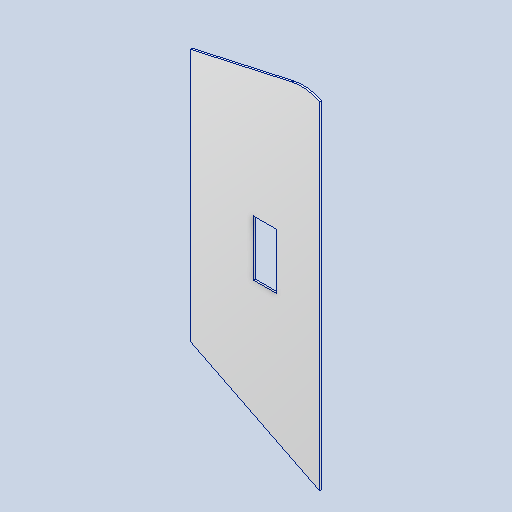
# Autodesk Inventor part: pokrywa lewa
Saved by Autodesk Inventor 2023 (Build 270158000, 158)
## iProperties
Created: 2022-10-11
Part Number: pokrywa lewa
Material: Aluminum 6061
Document SubType Name: Modeling
Designer: komputer
Density: 2.7 g/cm^3
Appearance: Aluminum - Flat
Author: komputer
Autodesk Inventor part; units mm, degrees
ref_plane "YZ Plane" through (0, 0, 0) normal (1, 0, 0) x (0, 1, 0)
ref_plane "XZ Plane" through (0, 0, 0) normal (0, 1, 0) x (-1, 0, 0)
ref_plane "XY Plane" through (0, 0, 0) normal (0, 0, 1) x (1, 0, 0)
sketch "Sketch1" plane through (0, 0, 0) normal (0, 0, 1) x (1, 0, 0)
  line L0 (7.5, 3.8038) -> (3.6225, 3.8038) projected
  arc A0 (1.9153, 4.762) -> (3.6225, 3.8038) centre (3.6225, 5.8038) ccw projected
  line L1 (1.9153, 4.762) -> (-2.2072, 11.517) projected
  arc A1 (-2.5, 12.5588) -> (-2.2072, 11.517) centre (-0.5, 12.5588) ccw projected
  line L2 (-2.5, 12.5588) -> (-2.5, 21.8038) projected
  arc A2 (-0.5, 23.8038) -> (-2.5, 21.8038) centre (-0.5, 21.8038) ccw projected
  line L3 (-0.5, 23.8038) -> (7.5, 23.8038) projected
  line L4 (7.5, 23.8038) -> (7.5, 3.8038) projected
  spline S0 degree 3 poles (-6.0485, -11.2843) (-6.0213, -11.0209) (-5.9428, -10.7653) (-5.6929, -10.2997) (-5.524, -10.094) (-5.1467, -9.7842) (-4.9505, -9.6718) (-4.5292, -9.5173) (-4.3073, -9.4763) (-4.0832, -9.4731) knots 0 0 0 0 0.079442 0.079442 0.158531 0.158531 0.225919 0.225919 0.293184 0.293184 0.293184 0.293184 projected
  line L5 (-6.0485, -11.2843) -> (-6.563, -16.2598) projected
  line L6 (-6.563, -16.2598) -> (-6.8849, -19.6266) projected
  arc A3 (-6.8849, -19.6266) -> (-5.7884, -21.6058) centre (-4.894, -19.817) ccw projected
  line L7 (17.5, -33.2499) -> (-5.7884, -21.6058) projected
  line L8 (17.5, 31.9794) -> (17.5, -33.2499) projected
  arc A4 (4.376, 33.2499) -> (17.5, 31.9794) centre (12.5, 48.7499) ccw projected
  arc A5 (-1.8324, 56.2463) -> (4.376, 33.2499) centre (12.5, 47.7794) ccw projected
  line L9 (-1.8324, 56.2463) -> (-17.5, 52.7794) projected
  line L10 (-17.5, 52.7794) -> (-17.5, 3.0185) projected
  ellipse E0 centre (-15.5, 3.0185) end of major axis (-15.5, 1.0011) minor radius 2 (-17.5, 3.0185) -> (-15.6888, 1.0101) ccw projected
  line L11 (-15.6888, 1.0101) -> (-3.1949, -0.1848) projected
  line L12 (-3.1949, -0.1848) -> (-4.0832, -9.4731) projected
  circle A6 centre (-12, 26.728) radius 1.25 projected
  circle A7 centre (5.3255, 26.728) radius 1.25 projected
  line L13 (-14, 9.2999) -> (-10, 9.2999) projected
  line L14 (-14, 15.6999) -> (-14, 9.2999) projected
  line L15 (-10, 15.6999) -> (-14, 15.6999) projected
  line L16 (-10, 9.2999) -> (-10, 15.6999) projected
  line L17 (13.7851, 6.0601) -> (9.7851, 6.0601) projected
  line L18 (13.7851, -0.3399) -> (13.7851, 6.0601) projected
  line L19 (9.7851, -0.3399) -> (13.7851, -0.3399) projected
  line L20 (9.7851, 6.0601) -> (9.7851, -0.3399) projected
  circle A8 centre (7.1425, -8.6154) radius 1.25 projected
  line L21 (17.5, -33.2499) -> (-17.5, -15.7501) projected
  line L22 (-17.5, -15.7501) -> (-17.5, -17.9862) projected
  line L23 (-17.5, -17.9862) -> (17.5, -35.486) projected
  line L24 (17.5, -35.486) -> (17.5, -33.2499) projected
  line L25 (-1.4649, 56.8397) -> (-18, 53.1809) projected
  line L26 (-18, 53.1809) -> (-18, -17.9862) projected
  line L27 (-18, -17.9862) -> (-17.5, -17.9862) projected
  line L28 (-17.5, -17.9862) -> (-17.5, 52.7794) projected
  line L29 (-17.5, 52.7794) -> (-1.8324, 56.2463) projected
  arc A9 (-1.4649, 56.8397) -> (-1.8324, 56.2463) centre (12.5, 47.7794) ccw projected
  line L30 (19.5, -37.0206) -> (19.5, 31.9794) projected
  line L31 (19.5, 31.9794) -> (17.5, 31.9794) projected
  line L32 (17.5, -37.0206) -> (17.5, 31.9794) projected
  line L33 (19.5, -37.0206) -> (17.5, -37.0206) projected
  circle A10 centre (12.5, 47.7794) radius 15.02 projected
  line L34 (-1.4649, 56.8397) -> (-11.9805, 54.5129)
  line L35 (-11.9805, 54.5129) -> (26.5324, 63.5095)
  line L36 (17.5, 31.9794) -> (17.5, 20.7849)
  line L37 (17.5, 20.7849) -> (17.5, 78.444)
  circle A11 centre (12.5, 47.7794) radius 12.1257
  line L38 (-17.5, -15.7501) -> (-17.5, 52.7794)
  line L39 (-1.8324, 56.2463) -> (11.2654, 59.1445)
  line L40 (11.2654, 59.1445) -> (26.5324, 62.5227)
  circle A12 centre (12.5, 47.7794) radius 11.3634
  line L41 (5.8925, 7.1892) -> (-0.5, 7.1892)
  line L42 (-0.5, 7.1892) -> (-0.5, 22.231)
  line L43 (-0.5, 22.231) -> (5.8925, 22.231)
  line L44 (5.8925, 22.231) -> (5.8925, 7.1892)
  point P0 (0, 0)
  point P1 (17.5, 57.9837)
  point P2 (10.0449, 58.8745)
  constraints: 22 end point, 4 point on line, 2 centre point, 2 coincident, 2 parallel, 2 tangent, 1 collinear, 1 horizontal, 1 perpendicular, 1 other
extrude "Extrusion1" add sketch "Sketch1" along normal blind 0.5 contours L0 A0 L1 L41 L44 L43 L42 A1 L2 A2 L3 L4 | L5 L6 A3 L21 L28 E0 L11 L12 S0 | S0 L12 L11 E0 L10 L9 A5 A4 L8 L7 A3 L6 L5 | L39 A10 L37 A4 A5 | L39 A11 L37 A10 | L39 A12 L37 A11 | A12 L37 | L14 L15 L16 L13 | L18 L19 L20 L17 picked at (9.8401, 51.5561)
sketch "Sketch2" plane through (0, 0, 0.5) normal (0, 0, 1) x (1, 0, 0)
  line L0 (17.5, -33.2499) -> (17.5, 57.9837) projected
  arc A0 (17.5, 57.9837) -> (10.0449, 58.8745) centre (12.5, 47.7794) ccw projected
  line L1 (10.0449, 58.8745) -> (-17.5, 52.7794) projected
  line L2 (-17.5, 52.7794) -> (-17.5, -15.7501) projected
  line L3 (-17.5, -15.7501) -> (17.5, -33.2499) projected
  circle A1 centre (-12, 26.728) radius 1.25 projected
  circle A2 centre (5.3255, 26.728) radius 1.25 projected
  circle A3 centre (7.1425, -8.6154) radius 1.25 projected
  line L4 (-0.5, 7.1892) -> (-0.5, 22.231) projected
  line L5 (-0.5, 22.231) -> (5.8925, 22.231) projected
  line L6 (5.8925, 22.231) -> (5.8925, 7.1892) projected
  line L7 (5.8925, 7.1892) -> (-0.5, 7.1892) projected
  point P0 (0, 0)
extrude "Extrusion2" add sketch "Sketch2" against normal blind 0.5 contours A1 | A2 | A3
body "Solid1"
